cube 2_v4 (Autodesk Fusion 360 design; units mm, degrees)
Autodesk Fusion 360 part; units mm, degrees
(part 1 of 2)
sketch "b  stock" plane through (0, 0, 0) normal (0, 0, 1) x (1, 0, 0)
  line L0 (0, 0) -> (50, 0)
  line L1 (50, 0) -> (50, 304.8)
  line L2 (50, 304.8) -> (0, 304.8)
  line L3 (0, 304.8) -> (0, 0)
extrude "b  stock body extrude" add sketch "b  stock" along normal blind 3.175 makes body 1
sketch "b  layout" plane through (0, 0, 0) normal (0, 0, 1) x (1, 0, 0)
  line L0 (0, 0) -> (48, 0)
  line L1 (48, 0) -> (48, 48)
  line L2 (48, 48) -> (0, 48)
  line L3 (0, 48) -> (0, 0)
  line L4 (0, 50.01) -> (48, 50.01)
  line L5 (48, 50.01) -> (48, 98.01)
  line L6 (48, 98.01) -> (0, 98.01)
  line L7 (0, 98.01) -> (0, 50.01)
  line L8 (0, 100.02) -> (48, 100.02)
  line L9 (48, 100.02) -> (48, 148.02)
  line L10 (48, 148.02) -> (0, 148.02)
  line L11 (0, 148.02) -> (0, 100.02)
  line L12 (0, 150.03) -> (48, 150.03)
  line L13 (48, 150.03) -> (48, 198.03)
  line L14 (48, 198.03) -> (0, 198.03)
  line L15 (0, 198.03) -> (0, 150.03)
  line L16 (0, 200.04) -> (48, 200.04)
  line L17 (48, 200.04) -> (48, 248.04)
  line L18 (48, 248.04) -> (0, 248.04)
  line L19 (0, 248.04) -> (0, 200.04)
  line L20 (0, 250.05) -> (48, 250.05)
  line L21 (48, 250.05) -> (48, 298.05)
  line L22 (48, 298.05) -> (0, 298.05)
  line L23 (0, 298.05) -> (0, 250.05)
sketch "b top lines" plane through (0, 0, 0) normal (0, 0, 1) x (1, 0, 0)
  line L0 (0, 0) -> (9.1, 0)
  line L1 (9.1, 0) -> (9.1, 3.175)
  line L2 (9.1, 3.175) -> (18.9, 3.175)
  line L3 (18.9, 3.175) -> (18.9, 0)
  line L4 (18.9, 0) -> (29.1, 0)
  line L5 (29.1, 0) -> (29.1, 3.175)
  line L6 (29.1, 3.175) -> (38.9, 3.175)
  line L7 (38.9, 3.175) -> (38.9, 0)
  line L8 (38.9, 0) -> (48, 0)
  line L9 (48, 0) -> (48, 9.1)
  line L10 (48, 9.1) -> (44.825, 9.1)
  line L11 (44.825, 9.1) -> (44.825, 18.9)
  line L12 (44.825, 18.9) -> (48, 18.9)
  line L13 (48, 18.9) -> (48, 29.1)
  line L14 (48, 29.1) -> (44.825, 29.1)
  line L15 (44.825, 29.1) -> (44.825, 38.9)
  line L16 (44.825, 38.9) -> (48, 38.9)
  line L17 (48, 38.9) -> (48, 48)
  line L18 (0, 48) -> (9.1, 48)
  line L19 (9.1, 48) -> (9.1, 44.825)
  line L20 (9.1, 44.825) -> (18.9, 44.825)
  line L21 (18.9, 44.825) -> (18.9, 48)
  line L22 (18.9, 48) -> (29.1, 48)
  line L23 (29.1, 48) -> (29.1, 44.825)
  line L24 (29.1, 44.825) -> (38.9, 44.825)
  line L25 (38.9, 44.825) -> (38.9, 48)
  line L26 (38.9, 48) -> (48, 48)
  line L27 (0, 0) -> (0, 9.1)
  line L28 (0, 9.1) -> (3.175, 9.1)
  line L29 (3.175, 9.1) -> (3.175, 18.9)
  line L30 (3.175, 18.9) -> (0, 18.9)
  line L31 (0, 18.9) -> (0, 29.1)
  line L32 (0, 29.1) -> (3.175, 29.1)
  line L33 (3.175, 29.1) -> (3.175, 38.9)
  line L34 (3.175, 38.9) -> (0, 38.9)
  line L35 (0, 38.9) -> (0, 48)
  dimension "d15" = 9.1
  dimension "d16" = 3.175
  dimension "d17" = 9.8
  dimension "d18" = 3.175
  dimension "d19" = 10.2
  dimension "d20" = 3.175
  dimension "d21" = 9.8
  dimension "d22" = 3.175
  dimension "d23" = 9.1
  dimension "d28" = 9.1
  dimension "d29" = 3.175
  dimension "d30" = 9.8
  dimension "d31" = 3.175
  dimension "d32" = 10.2
  dimension "d33" = 3.175
  dimension "d34" = 9.8
  dimension "d35" = 3.175
  dimension "d36" = 9.1
  dimension "d41" = 9.1
  dimension "d42" = 3.175
  dimension "d43" = 9.8
  dimension "d44" = 3.175
  dimension "d45" = 10.2
  dimension "d46" = 3.175
  dimension "d47" = 9.8
  dimension "d48" = 3.175
  dimension "d49" = 9.1
  dimension "d54" = 9.1
  dimension "d55" = 3.175
  dimension "d56" = 9.8
  dimension "d57" = 3.175
  dimension "d58" = 10.2
  dimension "d59" = 3.175
  dimension "d60" = 9.8
  dimension "d61" = 3.175
  dimension "d62" = 9.1
  constraint horizontal L0
  constraint vertical L1
  constraint horizontal L2
  constraint vertical L3
  constraint horizontal L4
  constraint vertical L5
  constraint horizontal L6
  constraint vertical L7
  constraint horizontal L8
  constraint vertical L9
  constraint horizontal L10
  constraint vertical L11
  constraint horizontal L12
  constraint vertical L13
  constraint horizontal L14
  constraint vertical L15
  constraint horizontal L16
  constraint vertical L17
  constraint horizontal L18
  constraint vertical L19
  constraint horizontal L20
  constraint vertical L21
  constraint horizontal L22
  constraint vertical L23
  constraint horizontal L24
  constraint vertical L25
  constraint horizontal L26
  constraint vertical L27
  constraint horizontal L28
  constraint vertical L29
  constraint horizontal L30
  constraint vertical L31
  constraint horizontal L32
  constraint vertical L33
  constraint horizontal L34
  constraint vertical L35
  measures "d15" distance of L0.start L0.end
  measures "d16" distance of L0.end L1.end
  measures "d17" distance of L1.end L2.end
  measures "d18" distance of L2.end L3.end
  measures "d19" distance of L3.end L4.end
  measures "d20" distance of L4.end L5.end
  measures "d21" distance of L5.end L6.end
  measures "d22" distance of L6.end L7.end
  measures "d23" distance of L7.end L8.end
  measures "d28" distance of L8.end L9.end
  measures "d29" distance of L9.end L10.end
  measures "d30" distance of L10.end L11.end
  measures "d31" distance of L11.end L12.end
  measures "d32" distance of L12.end L13.end
  measures "d33" distance of L13.end L14.end
  measures "d34" distance of L14.end L15.end
  measures "d35" distance of L15.end L16.end
  measures "d36" distance of L16.end L17.end
  measures "d41" distance of L18.start L18.end
  measures "d42" distance of L18.end L19.end
  measures "d43" distance of L19.end L20.end
  measures "d44" distance of L20.end L21.end
  measures "d45" distance of L21.end L22.end
  measures "d46" distance of L22.end L23.end
  measures "d47" distance of L23.end L24.end
  measures "d48" distance of L24.end L25.end
  measures "d49" distance of L17.end L25.end
  measures "d54" distance of L0.start L27.end
  measures "d55" distance of L27.end L28.end
  measures "d56" distance of L28.end L29.end
  measures "d57" distance of L29.end L30.end
  measures "d58" distance of L30.end L31.end
  measures "d59" distance of L31.end L32.end
  measures "d60" distance of L32.end L33.end
  measures "d61" distance of L33.end L34.end
  measures "d62" distance of L18.start L34.end
sketch "b top circles" plane through (0, 0, 0) normal (0, 0, 1) x (1, 0, 0)
  line L0 (0, 0) -> (48, 0)
  line L1 (48, 0) -> (48, 48)
  line L2 (48, 48) -> (0, 48)
  line L3 (0, 48) -> (0, 0)
  circle A0 centre (9.6906, 2.3644) radius 1.005
  circle A1 centre (18.3094, 2.3644) radius 1.005
  circle A2 centre (29.6906, 2.3644) radius 1.005
  circle A3 centre (38.3094, 2.3644) radius 1.005
  circle A4 centre (45.6356, 9.6906) radius 1.005
  circle A5 centre (45.6356, 18.3094) radius 1.005
  circle A6 centre (45.6356, 29.6906) radius 1.005
  circle A7 centre (45.6356, 38.3094) radius 1.005
  circle A8 centre (9.6906, 45.6356) radius 1.005
  circle A9 centre (18.3094, 45.6356) radius 1.005
  circle A10 centre (29.6906, 45.6356) radius 1.005
  circle A11 centre (38.3094, 45.6356) radius 1.005
  circle A12 centre (2.3644, 9.6906) radius 1.005
  circle A13 centre (2.3644, 18.3094) radius 1.005
  circle A14 centre (2.3644, 29.6906) radius 1.005
  circle A15 centre (2.3644, 38.3094) radius 1.005
  dimension "d24" = 2.01
  dimension "d25" = 2.01
  dimension "d26" = 2.01
  dimension "d27" = 2.01
  dimension "d37" = 2.01
  dimension "d38" = 2.01
  dimension "d39" = 2.01
  dimension "d40" = 2.01
  dimension "d50" = 2.01
  dimension "d51" = 2.01
  dimension "d52" = 2.01
  dimension "d53" = 2.01
  dimension "d63" = 2.01
  dimension "d64" = 2.01
  dimension "d65" = 2.01
  dimension "d66" = 2.01
  measures "d24" diameter of A0
  measures "d25" diameter of A1
  measures "d26" diameter of A2
  measures "d27" diameter of A3
  measures "d37" diameter of A4
  measures "d38" diameter of A5
  measures "d39" diameter of A6
  measures "d40" diameter of A7
  measures "d50" diameter of A8
  measures "d51" diameter of A9
  measures "d52" diameter of A10
  measures "d53" diameter of A11
  measures "d63" diameter of A12
  measures "d64" diameter of A13
  measures "d65" diameter of A14
  measures "d66" diameter of A15
extrude "b top lines body extrude" add sketch "b top lines" along normal blind 3.175 separate body makes body 2
extrude "b top circles extrude" add sketch "b top circles" along normal blind 3.175 separate body makes body 3
combine "b top lines final combine feature" operation intersect target body 2 tool bodies 3
sketch "b front lines" plane through (0, 0, 0) normal (0, 0, 1) x (1, 0, 0)
  line L0 (3.175, 53.185) -> (8.9, 53.185)
  line L1 (8.9, 53.185) -> (8.9, 50.01)
  line L2 (8.9, 50.01) -> (19.1, 50.01)
  line L3 (19.1, 50.01) -> (19.1, 53.185)
  line L4 (19.1, 53.185) -> (28.9, 53.185)
  line L5 (28.9, 53.185) -> (28.9, 50.01)
  line L6 (28.9, 50.01) -> (39.1, 50.01)
  line L7 (39.1, 50.01) -> (39.1, 53.185)
  line L8 (39.1, 53.185) -> (44.825, 53.185)
  line L9 (44.825, 53.185) -> (44.825, 58.91)
  line L10 (44.825, 58.91) -> (48, 58.91)
  line L11 (48, 58.91) -> (48, 69.11)
  line L12 (48, 69.11) -> (44.825, 69.11)
  line L13 (44.825, 69.11) -> (44.825, 78.91)
  line L14 (44.825, 78.91) -> (48, 78.91)
  line L15 (48, 78.91) -> (48, 89.11)
  line L16 (48, 89.11) -> (44.825, 89.11)
  line L17 (44.825, 89.11) -> (44.825, 94.835)
  line L18 (3.175, 94.835) -> (8.9, 94.835)
  line L19 (8.9, 94.835) -> (8.9, 98.01)
  line L20 (8.9, 98.01) -> (19.1, 98.01)
  line L21 (19.1, 98.01) -> (19.1, 94.835)
  line L22 (19.1, 94.835) -> (28.9, 94.835)
  line L23 (28.9, 94.835) -> (28.9, 98.01)
  line L24 (28.9, 98.01) -> (39.1, 98.01)
  line L25 (39.1, 98.01) -> (39.1, 94.835)
  line L26 (39.1, 94.835) -> (44.825, 94.835)
  line L27 (3.175, 53.185) -> (3.175, 58.91)
  line L28 (3.175, 58.91) -> (0, 58.91)
  line L29 (0, 58.91) -> (0, 69.11)
  line L30 (0, 69.11) -> (3.175, 69.11)
  line L31 (3.175, 69.11) -> (3.175, 78.91)
  line L32 (3.175, 78.91) -> (0, 78.91)
  line L33 (0, 78.91) -> (0, 89.11)
  line L34 (0, 89.11) -> (3.175, 89.11)
  line L35 (3.175, 89.11) -> (3.175, 94.835)
  dimension "d71" = 5.725
  dimension "d72" = 3.175
  dimension "d73" = 10.2
  dimension "d74" = 3.175
  dimension "d75" = 9.8
  dimension "d76" = 3.175
  dimension "d77" = 10.2
  dimension "d78" = 3.175
  dimension "d79" = 5.725
  dimension "d84" = 5.725
  dimension "d85" = 3.175
  dimension "d86" = 10.2
  dimension "d87" = 3.175
  dimension "d88" = 9.8
  dimension "d89" = 3.175
  dimension "d90" = 10.2
  dimension "d91" = 3.175
  dimension "d92" = 5.725
  dimension "d97" = 5.725
  dimension "d98" = 3.175
  dimension "d99" = 10.2
  dimension "d100" = 3.175
  dimension "d101" = 9.8
  dimension "d102" = 3.175
  dimension "d103" = 10.2
  dimension "d104" = 3.175
  dimension "d105" = 5.725
  dimension "d110" = 5.725
  dimension "d111" = 3.175
  dimension "d112" = 10.2
  dimension "d113" = 3.175
  dimension "d114" = 9.8
  dimension "d115" = 3.175
  dimension "d116" = 10.2
  dimension "d117" = 3.175
  dimension "d118" = 5.725
  constraint horizontal L0
  constraint vertical L1
  constraint horizontal L2
  constraint vertical L3
  constraint horizontal L4
  constraint vertical L5
  constraint horizontal L6
  constraint vertical L7
  constraint horizontal L8
  constraint vertical L9
  constraint horizontal L10
  constraint vertical L11
  constraint horizontal L12
  constraint vertical L13
  constraint horizontal L14
  constraint vertical L15
  constraint horizontal L16
  constraint vertical L17
  constraint horizontal L18
  constraint vertical L19
  constraint horizontal L20
  constraint vertical L21
  constraint horizontal L22
  constraint vertical L23
  constraint horizontal L24
  constraint vertical L25
  constraint horizontal L26
  constraint vertical L27
  constraint horizontal L28
  constraint vertical L29
  constraint horizontal L30
  constraint vertical L31
  constraint horizontal L32
  constraint vertical L33
  constraint horizontal L34
  constraint vertical L35
  measures "d71" distance of L0.start L0.end
  measures "d72" distance of L0.end L1.end
  measures "d73" distance of L1.end L2.end
  measures "d74" distance of L2.end L3.end
  measures "d75" distance of L3.end L4.end
  measures "d76" distance of L4.end L5.end
  measures "d77" distance of L5.end L6.end
  measures "d78" distance of L6.end L7.end
  measures "d79" distance of L7.end L8.end
  measures "d84" distance of L8.end L9.end
  measures "d85" distance of L9.end L10.end
  measures "d86" distance of L10.end L11.end
  measures "d87" distance of L11.end L12.end
  measures "d88" distance of L12.end L13.end
  measures "d89" distance of L13.end L14.end
  measures "d90" distance of L14.end L15.end
  measures "d91" distance of L15.end L16.end
  measures "d92" distance of L16.end L17.end
  measures "d97" distance of L18.start L18.end
  measures "d98" distance of L18.end L19.end
  measures "d99" distance of L19.end L20.end
  measures "d100" distance of L20.end L21.end
  measures "d101" distance of L21.end L22.end
  measures "d102" distance of L22.end L23.end
  measures "d103" distance of L23.end L24.end
  measures "d104" distance of L24.end L25.end
  measures "d105" distance of L17.end L25.end
  measures "d110" distance of L0.start L27.end
  measures "d111" distance of L27.end L28.end
  measures "d112" distance of L28.end L29.end
  measures "d113" distance of L29.end L30.end
  measures "d114" distance of L30.end L31.end
  measures "d115" distance of L31.end L32.end
  measures "d116" distance of L32.end L33.end
  measures "d117" distance of L33.end L34.end
  measures "d118" distance of L18.start L34.end
sketch "b front circles" plane through (0, 0, 0) normal (0, 0, 1) x (1, 0, 0)
  line L0 (0, 50.01) -> (48, 50.01)
  line L1 (48, 50.01) -> (48, 98.01)
  line L2 (48, 98.01) -> (0, 98.01)
  line L3 (0, 98.01) -> (0, 50.01)
  circle A0 centre (8.3094, 52.3744) radius 1.005
  circle A1 centre (19.6906, 52.3744) radius 1.005
  circle A2 centre (28.3094, 52.3744) radius 1.005
  circle A3 centre (39.6906, 52.3744) radius 1.005
  circle A4 centre (45.6356, 58.3194) radius 1.005
  circle A5 centre (45.6356, 69.7006) radius 1.005
  circle A6 centre (45.6356, 78.3194) radius 1.005
  circle A7 centre (45.6356, 89.7006) radius 1.005
  circle A8 centre (8.3094, 95.6456) radius 1.005
  circle A9 centre (19.6906, 95.6456) radius 1.005
  circle A10 centre (28.3094, 95.6456) radius 1.005
  circle A11 centre (39.6906, 95.6456) radius 1.005
  circle A12 centre (2.3644, 58.3194) radius 1.005
  circle A13 centre (2.3644, 69.7006) radius 1.005
  circle A14 centre (2.3644, 78.3194) radius 1.005
  circle A15 centre (2.3644, 89.7006) radius 1.005
  dimension "d80" = 2.01
  dimension "d81" = 2.01
  dimension "d82" = 2.01
  dimension "d83" = 2.01
  dimension "d93" = 2.01
  dimension "d94" = 2.01
  dimension "d95" = 2.01
  dimension "d96" = 2.01
  dimension "d106" = 2.01
  dimension "d107" = 2.01
  dimension "d108" = 2.01
  dimension "d109" = 2.01
  dimension "d119" = 2.01
  dimension "d120" = 2.01
  dimension "d121" = 2.01
  dimension "d122" = 2.01
  measures "d80" diameter of A0
  measures "d81" diameter of A1
  measures "d82" diameter of A2
  measures "d83" diameter of A3
  measures "d93" diameter of A4
  measures "d94" diameter of A5
  measures "d95" diameter of A6
  measures "d96" diameter of A7
  measures "d106" diameter of A8
  measures "d107" diameter of A9
  measures "d108" diameter of A10
  measures "d109" diameter of A11
  measures "d119" diameter of A12
  measures "d120" diameter of A13
  measures "d121" diameter of A14
  measures "d122" diameter of A15
extrude "b front lines body extrude" add sketch "b front lines" along normal blind 3.175 separate body makes body 4
extrude "b front circles extrude" add sketch "b front circles" along normal blind 3.175 separate body makes body 5
combine "b front lines final combine feature" operation intersect target body 4 tool bodies 5
sketch "b back lines" plane through (0, 0, 0) normal (0, 0, 1) x (1, 0, 0)
  line L0 (3.175, 103.195) -> (8.9, 103.195)
  line L1 (8.9, 103.195) -> (8.9, 100.02)
  line L2 (8.9, 100.02) -> (19.1, 100.02)
  line L3 (19.1, 100.02) -> (19.1, 103.195)
  line L4 (19.1, 103.195) -> (28.9, 103.195)
  line L5 (28.9, 103.195) -> (28.9, 100.02)
  line L6 (28.9, 100.02) -> (39.1, 100.02)
  line L7 (39.1, 100.02) -> (39.1, 103.195)
  line L8 (39.1, 103.195) -> (44.825, 103.195)
  line L9 (44.825, 103.195) -> (44.825, 108.92)
  line L10 (44.825, 108.92) -> (48, 108.92)
  line L11 (48, 108.92) -> (48, 119.12)
  line L12 (48, 119.12) -> (44.825, 119.12)
  line L13 (44.825, 119.12) -> (44.825, 128.92)
  line L14 (44.825, 128.92) -> (48, 128.92)
  line L15 (48, 128.92) -> (48, 139.12)
  line L16 (48, 139.12) -> (44.825, 139.12)
  line L17 (44.825, 139.12) -> (44.825, 144.845)
  line L18 (3.175, 144.845) -> (8.9, 144.845)
  line L19 (8.9, 144.845) -> (8.9, 148.02)
  line L20 (8.9, 148.02) -> (19.1, 148.02)
  line L21 (19.1, 148.02) -> (19.1, 144.845)
  line L22 (19.1, 144.845) -> (28.9, 144.845)
  line L23 (28.9, 144.845) -> (28.9, 148.02)
  line L24 (28.9, 148.02) -> (39.1, 148.02)
  line L25 (39.1, 148.02) -> (39.1, 144.845)
  line L26 (39.1, 144.845) -> (44.825, 144.845)
  line L27 (3.175, 103.195) -> (3.175, 108.92)
  line L28 (3.175, 108.92) -> (0, 108.92)
  line L29 (0, 108.92) -> (0, 119.12)
  line L30 (0, 119.12) -> (3.175, 119.12)
  line L31 (3.175, 119.12) -> (3.175, 128.92)
  line L32 (3.175, 128.92) -> (0, 128.92)
  line L33 (0, 128.92) -> (0, 139.12)
  line L34 (0, 139.12) -> (3.175, 139.12)
  line L35 (3.175, 139.12) -> (3.175, 144.845)
  dimension "d127" = 5.725
  dimension "d128" = 3.175
  dimension "d129" = 10.2
  dimension "d130" = 3.175
  dimension "d131" = 9.8
  dimension "d132" = 3.175
  dimension "d133" = 10.2
  dimension "d134" = 3.175
  dimension "d135" = 5.725
  dimension "d140" = 5.725
  dimension "d141" = 3.175
  dimension "d142" = 10.2
  dimension "d143" = 3.175
  dimension "d144" = 9.8
  dimension "d145" = 3.175
  dimension "d146" = 10.2
  dimension "d147" = 3.175
  dimension "d148" = 5.725
  dimension "d153" = 5.725
  dimension "d154" = 3.175
  dimension "d155" = 10.2
  dimension "d156" = 3.175
  dimension "d157" = 9.8
  dimension "d158" = 3.175
  dimension "d159" = 10.2
  dimension "d160" = 3.175
  dimension "d161" = 5.725
  dimension "d166" = 5.725
  dimension "d167" = 3.175
  dimension "d168" = 10.2
  dimension "d169" = 3.175
  dimension "d170" = 9.8
  dimension "d171" = 3.175
  dimension "d172" = 10.2
  dimension "d173" = 3.175
  dimension "d174" = 5.725
  constraint horizontal L0
  constraint vertical L1
  constraint horizontal L2
  constraint vertical L3
  constraint horizontal L4
  constraint vertical L5
  constraint horizontal L6
  constraint vertical L7
  constraint horizontal L8
  constraint vertical L9
  constraint horizontal L10
  constraint vertical L11
  constraint horizontal L12
  constraint vertical L13
  constraint horizontal L14
  constraint vertical L15
  constraint horizontal L16
  constraint vertical L17
  constraint horizontal L18
  constraint vertical L19
  constraint horizontal L20
  constraint vertical L21
  constraint horizontal L22
  constraint vertical L23
  constraint horizontal L24
  constraint vertical L25
  constraint horizontal L26
  constraint vertical L27
  constraint horizontal L28
  constraint vertical L29
  constraint horizontal L30
  constraint vertical L31
  constraint horizontal L32
  constraint vertical L33
  constraint horizontal L34
  constraint vertical L35
  measures "d127" distance of L0.start L0.end
  measures "d128" distance of L0.end L1.end
  measures "d129" distance of L1.end L2.end
  measures "d130" distance of L2.end L3.end
  measures "d131" distance of L3.end L4.end
  measures "d132" distance of L4.end L5.end
  measures "d133" distance of L5.end L6.end
  measures "d134" distance of L6.end L7.end
  measures "d135" distance of L7.end L8.end
  measures "d140" distance of L8.end L9.end
  measures "d141" distance of L9.end L10.end
  measures "d142" distance of L10.end L11.end
  measures "d143" distance of L11.end L12.end
  measures "d144" distance of L12.end L13.end
  measures "d145" distance of L13.end L14.end
  measures "d146" distance of L14.end L15.end
  measures "d147" distance of L15.end L16.end
  measures "d148" distance of L16.end L17.end
  measures "d153" distance of L18.start L18.end
  measures "d154" distance of L18.end L19.end
  measures "d155" distance of L19.end L20.end
  measures "d156" distance of L20.end L21.end
  measures "d157" distance of L21.end L22.end
  measures "d158" distance of L22.end L23.end
  measures "d159" distance of L23.end L24.end
  measures "d160" distance of L24.end L25.end
  measures "d161" distance of L17.end L25.end
  measures "d166" distance of L0.start L27.end
  measures "d167" distance of L27.end L28.end
  measures "d168" distance of L28.end L29.end
  measures "d169" distance of L29.end L30.end
  measures "d170" distance of L30.end L31.end
  measures "d171" distance of L31.end L32.end
  measures "d172" distance of L32.end L33.end
  measures "d173" distance of L33.end L34.end
  measures "d174" distance of L18.start L34.end
sketch "b back circles" plane through (0, 0, 0) normal (0, 0, 1) x (1, 0, 0)
  line L0 (0, 100.02) -> (48, 100.02)
  line L1 (48, 100.02) -> (48, 148.02)
  line L2 (48, 148.02) -> (0, 148.02)
  line L3 (0, 148.02) -> (0, 100.02)
  circle A0 centre (8.3094, 102.3844) radius 1.005
  circle A1 centre (19.6906, 102.3844) radius 1.005
  circle A2 centre (28.3094, 102.3844) radius 1.005
  circle A3 centre (39.6906, 102.3844) radius 1.005
  circle A4 centre (45.6356, 108.3294) radius 1.005
  circle A5 centre (45.6356, 119.7106) radius 1.005
  circle A6 centre (45.6356, 128.3294) radius 1.005
  circle A7 centre (45.6356, 139.7106) radius 1.005
  circle A8 centre (8.3094, 145.6556) radius 1.005
  circle A9 centre (19.6906, 145.6556) radius 1.005
  circle A10 centre (28.3094, 145.6556) radius 1.005
  circle A11 centre (39.6906, 145.6556) radius 1.005
  circle A12 centre (2.3644, 108.3294) radius 1.005
  circle A13 centre (2.3644, 119.7106) radius 1.005
  circle A14 centre (2.3644, 128.3294) radius 1.005
  circle A15 centre (2.3644, 139.7106) radius 1.005
  dimension "d136" = 2.01
  dimension "d137" = 2.01
  dimension "d138" = 2.01
  dimension "d139" = 2.01
  dimension "d149" = 2.01
  dimension "d150" = 2.01
  dimension "d151" = 2.01
  dimension "d152" = 2.01
  dimension "d162" = 2.01
  dimension "d163" = 2.01
  dimension "d164" = 2.01
  dimension "d165" = 2.01
  dimension "d175" = 2.01
  dimension "d176" = 2.01
  dimension "d177" = 2.01
  dimension "d178" = 2.01
  measures "d136" diameter of A0
  measures "d137" diameter of A1
  measures "d138" diameter of A2
  measures "d139" diameter of A3
  measures "d149" diameter of A4
  measures "d150" diameter of A5
  measures "d151" diameter of A6
  measures "d152" diameter of A7
  measures "d162" diameter of A8
  measures "d163" diameter of A9
  measures "d164" diameter of A10
  measures "d165" diameter of A11
  measures "d175" diameter of A12
  measures "d176" diameter of A13
  measures "d177" diameter of A14
  measures "d178" diameter of A15
extrude "b back lines body extrude" add sketch "b back lines" along normal blind 3.175 separate body makes body 6
extrude "b back circles extrude" add sketch "b back circles" along normal blind 3.175 separate body makes body 7
combine "b back lines final combine feature" operation intersect target body 6 tool bodies 7
sketch "b left lines" plane through (0, 0, 0) normal (0, 0, 1) x (1, 0, 0)
  line L0 (3.175, 150.03) -> (9.1, 150.03)
  line L1 (9.1, 150.03) -> (9.1, 153.205)
  line L2 (9.1, 153.205) -> (18.9, 153.205)
  line L3 (18.9, 153.205) -> (18.9, 150.03)
  line L4 (18.9, 150.03) -> (29.1, 150.03)
  line L5 (29.1, 150.03) -> (29.1, 153.205)
  line L6 (29.1, 153.205) -> (38.9, 153.205)
  line L7 (38.9, 153.205) -> (38.9, 150.03)
  line L8 (38.9, 150.03) -> (44.825, 150.03)
  line L9 (44.825, 150.03) -> (44.825, 158.93)
  line L10 (44.825, 158.93) -> (48, 158.93)
  line L11 (48, 158.93) -> (48, 169.13)
  line L12 (48, 169.13) -> (44.825, 169.13)
  line L13 (44.825, 169.13) -> (44.825, 178.93)
  line L14 (44.825, 178.93) -> (48, 178.93)
  line L15 (48, 178.93) -> (48, 189.13)
  line L16 (48, 189.13) -> (44.825, 189.13)
  line L17 (44.825, 189.13) -> (44.825, 198.03)
  line L18 (3.175, 198.03) -> (9.1, 198.03)
  line L19 (9.1, 198.03) -> (9.1, 194.855)
  line L20 (9.1, 194.855) -> (18.9, 194.855)
  line L21 (18.9, 194.855) -> (18.9, 198.03)
  line L22 (18.9, 198.03) -> (29.1, 198.03)
  line L23 (29.1, 198.03) -> (29.1, 194.855)
  line L24 (29.1, 194.855) -> (38.9, 194.855)
  line L25 (38.9, 194.855) -> (38.9, 198.03)
  line L26 (38.9, 198.03) -> (44.825, 198.03)
  line L27 (3.175, 150.03) -> (3.175, 158.93)
  line L28 (3.175, 158.93) -> (0, 158.93)
  line L29 (0, 158.93) -> (0, 169.13)
  line L30 (0, 169.13) -> (3.175, 169.13)
  line L31 (3.175, 169.13) -> (3.175, 178.93)
  line L32 (3.175, 178.93) -> (0, 178.93)
  line L33 (0, 178.93) -> (0, 189.13)
  line L34 (0, 189.13) -> (3.175, 189.13)
  line L35 (3.175, 189.13) -> (3.175, 198.03)
  dimension "d183" = 5.925
  dimension "d184" = 3.175
  dimension "d185" = 9.8
  dimension "d186" = 3.175
  dimension "d187" = 10.2
  dimension "d188" = 3.175
  dimension "d189" = 9.8
  dimension "d190" = 3.175
  dimension "d191" = 5.925
  dimension "d196" = 8.9
  dimension "d197" = 3.175
  dimension "d198" = 10.2
  dimension "d199" = 3.175
  dimension "d200" = 9.8
  dimension "d201" = 3.175
  dimension "d202" = 10.2
  dimension "d203" = 3.175
  dimension "d204" = 8.9
  dimension "d209" = 5.925
  dimension "d210" = 3.175
  dimension "d211" = 9.8
  dimension "d212" = 3.175
  dimension "d213" = 10.2
  dimension "d214" = 3.175
  dimension "d215" = 9.8
  dimension "d216" = 3.175
  dimension "d217" = 5.925
  dimension "d222" = 8.9
  dimension "d223" = 3.175
  dimension "d224" = 10.2
  dimension "d225" = 3.175
  dimension "d226" = 9.8
  dimension "d227" = 3.175
  dimension "d228" = 10.2
  dimension "d229" = 3.175
  dimension "d230" = 8.9
  constraint horizontal L0
  constraint vertical L1
  constraint horizontal L2
  constraint vertical L3
  constraint horizontal L4
  constraint vertical L5
  constraint horizontal L6
  constraint vertical L7
  constraint horizontal L8
  constraint vertical L9
  constraint horizontal L10
  constraint vertical L11
  constraint horizontal L12
  constraint vertical L13
  constraint horizontal L14
  constraint vertical L15
  constraint horizontal L16
  constraint vertical L17
  constraint horizontal L18
  constraint vertical L19
  constraint horizontal L20
  constraint vertical L21
  constraint horizontal L22
  constraint vertical L23
  constraint horizontal L24
  constraint vertical L25
  constraint horizontal L26
  constraint vertical L27
  constraint horizontal L28
  constraint vertical L29
  constraint horizontal L30
  constraint vertical L31
  constraint horizontal L32
  constraint vertical L33
  constraint horizontal L34
  constraint vertical L35
  measures "d183" distance of L0.start L0.end
  measures "d184" distance of L0.end L1.end
  measures "d185" distance of L1.end L2.end
  measures "d186" distance of L2.end L3.end
  measures "d187" distance of L3.end L4.end
  measures "d188" distance of L4.end L5.end
  measures "d189" distance of L5.end L6.end
  measures "d190" distance of L6.end L7.end
  measures "d191" distance of L7.end L8.end
  measures "d196" distance of L8.end L9.end
  measures "d197" distance of L9.end L10.end
  measures "d198" distance of L10.end L11.end
  measures "d199" distance of L11.end L12.end
  measures "d200" distance of L12.end L13.end
  measures "d201" distance of L13.end L14.end
  measures "d202" distance of L14.end L15.end
  measures "d203" distance of L15.end L16.end
  measures "d204" distance of L16.end L17.end
  measures "d209" distance of L18.start L18.end
  measures "d210" distance of L18.end L19.end
  measures "d211" distance of L19.end L20.end
  measures "d212" distance of L20.end L21.end
  measures "d213" distance of L21.end L22.end
  measures "d214" distance of L22.end L23.end
  measures "d215" distance of L23.end L24.end
  measures "d216" distance of L24.end L25.end
  measures "d217" distance of L17.end L25.end
  measures "d222" distance of L0.start L27.end
  measures "d223" distance of L27.end L28.end
  measures "d224" distance of L28.end L29.end
  measures "d225" distance of L29.end L30.end
  measures "d226" distance of L30.end L31.end
  measures "d227" distance of L31.end L32.end
  measures "d228" distance of L32.end L33.end
  measures "d229" distance of L33.end L34.end
  measures "d230" distance of L18.start L34.end
sketch "b left circles" plane through (0, 0, 0) normal (0, 0, 1) x (1, 0, 0)
  line L0 (0, 150.03) -> (48, 150.03)
  line L1 (48, 150.03) -> (48, 198.03)
  line L2 (48, 198.03) -> (0, 198.03)
  line L3 (0, 198.03) -> (0, 150.03)
  circle A0 centre (9.6906, 152.3944) radius 1.005
  circle A1 centre (18.3094, 152.3944) radius 1.005
  circle A2 centre (29.6906, 152.3944) radius 1.005
  circle A3 centre (38.3094, 152.3944) radius 1.005
  circle A4 centre (45.6356, 158.3394) radius 1.005
  circle A5 centre (45.6356, 169.7206) radius 1.005
  circle A6 centre (45.6356, 178.3394) radius 1.005
  circle A7 centre (45.6356, 189.7206) radius 1.005
  circle A8 centre (9.6906, 195.6656) radius 1.005
  circle A9 centre (18.3094, 195.6656) radius 1.005
  circle A10 centre (29.6906, 195.6656) radius 1.005
  circle A11 centre (38.3094, 195.6656) radius 1.005
  circle A12 centre (2.3644, 158.3394) radius 1.005
  circle A13 centre (2.3644, 169.7206) radius 1.005
  circle A14 centre (2.3644, 178.3394) radius 1.005
  circle A15 centre (2.3644, 189.7206) radius 1.005
  dimension "d192" = 2.01
  dimension "d193" = 2.01
  dimension "d194" = 2.01
  dimension "d195" = 2.01
  dimension "d205" = 2.01
  dimension "d206" = 2.01
  dimension "d207" = 2.01
  dimension "d208" = 2.01
  dimension "d218" = 2.01
  dimension "d219" = 2.01
  dimension "d220" = 2.01
  dimension "d221" = 2.01
  dimension "d231" = 2.01
  dimension "d232" = 2.01
  dimension "d233" = 2.01
  dimension "d234" = 2.01
  measures "d192" diameter of A0
  measures "d193" diameter of A1
  measures "d194" diameter of A2
  measures "d195" diameter of A3
  measures "d205" diameter of A4
  measures "d206" diameter of A5
  measures "d207" diameter of A6
  measures "d208" diameter of A7
  measures "d218" diameter of A8
  measures "d219" diameter of A9
  measures "d220" diameter of A10
  measures "d221" diameter of A11
  measures "d231" diameter of A12
  measures "d232" diameter of A13
  measures "d233" diameter of A14
  measures "d234" diameter of A15
extrude "b left lines body extrude" add sketch "b left lines" along normal blind 3.175 separate body makes body 8
extrude "b left circles extrude" add sketch "b left circles" along normal blind 3.175 separate body makes body 9
combine "b left lines final combine feature" operation intersect target body 8 tool bodies 9
sketch "b right lines" plane through (0, 0, 0) normal (0, 0, 1) x (1, 0, 0)
  line L0 (3.175, 200.04) -> (9.1, 200.04)
  line L1 (9.1, 200.04) -> (9.1, 203.215)
  line L2 (9.1, 203.215) -> (18.9, 203.215)
  line L3 (18.9, 203.215) -> (18.9, 200.04)
  line L4 (18.9, 200.04) -> (29.1, 200.04)
  line L5 (29.1, 200.04) -> (29.1, 203.215)
  line L6 (29.1, 203.215) -> (38.9, 203.215)
  line L7 (38.9, 203.215) -> (38.9, 200.04)
  line L8 (38.9, 200.04) -> (44.825, 200.04)
  line L9 (44.825, 200.04) -> (44.825, 208.94)
  line L10 (44.825, 208.94) -> (48, 208.94)
  line L11 (48, 208.94) -> (48, 219.14)
  line L12 (48, 219.14) -> (44.825, 219.14)
  line L13 (44.825, 219.14) -> (44.825, 228.94)
  line L14 (44.825, 228.94) -> (48, 228.94)
  line L15 (48, 228.94) -> (48, 239.14)
  line L16 (48, 239.14) -> (44.825, 239.14)
  line L17 (44.825, 239.14) -> (44.825, 248.04)
  line L18 (3.175, 248.04) -> (9.1, 248.04)
  line L19 (9.1, 248.04) -> (9.1, 244.865)
  line L20 (9.1, 244.865) -> (18.9, 244.865)
  line L21 (18.9, 244.865) -> (18.9, 248.04)
  line L22 (18.9, 248.04) -> (29.1, 248.04)
  line L23 (29.1, 248.04) -> (29.1, 244.865)
  line L24 (29.1, 244.865) -> (38.9, 244.865)
  line L25 (38.9, 244.865) -> (38.9, 248.04)
  line L26 (38.9, 248.04) -> (44.825, 248.04)
  line L27 (3.175, 200.04) -> (3.175, 208.94)
  line L28 (3.175, 208.94) -> (0, 208.94)
  line L29 (0, 208.94) -> (0, 219.14)
  line L30 (0, 219.14) -> (3.175, 219.14)
  line L31 (3.175, 219.14) -> (3.175, 228.94)
  line L32 (3.175, 228.94) -> (0, 228.94)
  line L33 (0, 228.94) -> (0, 239.14)
  line L34 (0, 239.14) -> (3.175, 239.14)
  line L35 (3.175, 239.14) -> (3.175, 248.04)
  dimension "d239" = 5.925
  dimension "d240" = 3.175
  dimension "d241" = 9.8
  dimension "d242" = 3.175
  dimension "d243" = 10.2
  dimension "d244" = 3.175
  dimension "d245" = 9.8
  dimension "d246" = 3.175
  dimension "d247" = 5.925
  dimension "d252" = 8.9
  dimension "d253" = 3.175
  dimension "d254" = 10.2
  dimension "d255" = 3.175
  dimension "d256" = 9.8
  dimension "d257" = 3.175
  dimension "d258" = 10.2
  dimension "d259" = 3.175
  dimension "d260" = 8.9
  dimension "d265" = 5.925
  dimension "d266" = 3.175
  dimension "d267" = 9.8
  dimension "d268" = 3.175
  dimension "d269" = 10.2
  dimension "d270" = 3.175
  dimension "d271" = 9.8
  dimension "d272" = 3.175
  dimension "d273" = 5.925
  dimension "d278" = 8.9
  dimension "d279" = 3.175
  dimension "d280" = 10.2
  dimension "d281" = 3.175
  dimension "d282" = 9.8
  dimension "d283" = 3.175
  dimension "d284" = 10.2
  dimension "d285" = 3.175
  dimension "d286" = 8.9
  constraint horizontal L0
  constraint vertical L1
  constraint horizontal L2
  constraint vertical L3
  constraint horizontal L4
  constraint vertical L5
  constraint horizontal L6
  constraint vertical L7
  constraint horizontal L8
  constraint vertical L9
  constraint horizontal L10
  constraint vertical L11
  constraint horizontal L12
  constraint vertical L13
  constraint horizontal L14
  constraint vertical L15
  constraint horizontal L16
  constraint vertical L17
  constraint horizontal L18
  constraint vertical L19
  constraint horizontal L20
  constraint vertical L21
  constraint horizontal L22
  constraint vertical L23
  constraint horizontal L24
  constraint vertical L25
  constraint horizontal L26
  constraint vertical L27
  constraint horizontal L28
  constraint vertical L29
  constraint horizontal L30
  constraint vertical L31
  constraint horizontal L32
  constraint vertical L33
  constraint horizontal L34
  constraint vertical L35
  measures "d239" distance of L0.start L0.end
  measures "d240" distance of L0.end L1.end
  measures "d241" distance of L1.end L2.end
  measures "d242" distance of L2.end L3.end
  measures "d243" distance of L3.end L4.end
  measures "d244" distance of L4.end L5.end
  measures "d245" distance of L5.end L6.end
  measures "d246" distance of L6.end L7.end
  measures "d247" distance of L7.end L8.end
  measures "d252" distance of L8.end L9.end
  measures "d253" distance of L9.end L10.end
  measures "d254" distance of L10.end L11.end
  measures "d255" distance of L11.end L12.end
  measures "d256" distance of L12.end L13.end
  measures "d257" distance of L13.end L14.end
  measures "d258" distance of L14.end L15.end
  measures "d259" distance of L15.end L16.end
  measures "d260" distance of L16.end L17.end
  measures "d265" distance of L18.start L18.end
  measures "d266" distance of L18.end L19.end
  measures "d267" distance of L19.end L20.end
  measures "d268" distance of L20.end L21.end
  measures "d269" distance of L21.end L22.end
  measures "d270" distance of L22.end L23.end
  measures "d271" distance of L23.end L24.end
  measures "d272" distance of L24.end L25.end
  measures "d273" distance of L17.end L25.end
  measures "d278" distance of L0.start L27.end
  measures "d279" distance of L27.end L28.end
  measures "d280" distance of L28.end L29.end
  measures "d281" distance of L29.end L30.end
  measures "d282" distance of L30.end L31.end
  measures "d283" distance of L31.end L32.end
  measures "d284" distance of L32.end L33.end
  measures "d285" distance of L33.end L34.end
  measures "d286" distance of L18.start L34.end
sketch "b right circles" plane through (0, 0, 0) normal (0, 0, 1) x (1, 0, 0)
  line L0 (0, 200.04) -> (48, 200.04)
  line L1 (48, 200.04) -> (48, 248.04)
  line L2 (48, 248.04) -> (0, 248.04)
  line L3 (0, 248.04) -> (0, 200.04)
  circle A0 centre (9.6906, 202.4044) radius 1.005
  circle A1 centre (18.3094, 202.4044) radius 1.005
  circle A2 centre (29.6906, 202.4044) radius 1.005
  circle A3 centre (38.3094, 202.4044) radius 1.005
  circle A4 centre (45.6356, 208.3494) radius 1.005
  circle A5 centre (45.6356, 219.7306) radius 1.005
  circle A6 centre (45.6356, 228.3494) radius 1.005
  circle A7 centre (45.6356, 239.7306) radius 1.005
  circle A8 centre (9.6906, 245.6756) radius 1.005
  circle A9 centre (18.3094, 245.6756) radius 1.005
  circle A10 centre (29.6906, 245.6756) radius 1.005
  circle A11 centre (38.3094, 245.6756) radius 1.005
  circle A12 centre (2.3644, 208.3494) radius 1.005
  circle A13 centre (2.3644, 219.7306) radius 1.005
  circle A14 centre (2.3644, 228.3494) radius 1.005
  circle A15 centre (2.3644, 239.7306) radius 1.005
  dimension "d248" = 2.01
  dimension "d249" = 2.01
  dimension "d250" = 2.01
  dimension "d251" = 2.01
  dimension "d261" = 2.01
  dimension "d262" = 2.01
  dimension "d263" = 2.01
  dimension "d264" = 2.01
  dimension "d274" = 2.01
  dimension "d275" = 2.01
  dimension "d276" = 2.01
  dimension "d277" = 2.01
  dimension "d287" = 2.01
  dimension "d288" = 2.01
  dimension "d289" = 2.01
  dimension "d290" = 2.01
  measures "d248" diameter of A0
  measures "d249" diameter of A1
  measures "d250" diameter of A2
  measures "d251" diameter of A3
  measures "d261" diameter of A4
  measures "d262" diameter of A5
  measures "d263" diameter of A6
  measures "d264" diameter of A7
  measures "d274" diameter of A8
  measures "d275" diameter of A9
  measures "d276" diameter of A10
  measures "d277" diameter of A11
  measures "d287" diameter of A12
  measures "d288" diameter of A13
  measures "d289" diameter of A14
  measures "d290" diameter of A15
extrude "b right lines body extrude" add sketch "b right lines" along normal blind 3.175 separate body makes body 10
extrude "b right circles extrude" add sketch "b right circles" along normal blind 3.175 separate body makes body 11
combine "b right lines final combine feature" operation intersect target body 10 tool bodies 11
sketch "b bottom lines" plane through (0, 0, 0) normal (0, 0, 1) x (1, 0, 0)
  line L0 (0, 250.05) -> (9.1, 250.05)
  line L1 (9.1, 250.05) -> (9.1, 253.225)
  line L2 (9.1, 253.225) -> (18.9, 253.225)
  line L3 (18.9, 253.225) -> (18.9, 250.05)
  line L4 (18.9, 250.05) -> (29.1, 250.05)
  line L5 (29.1, 250.05) -> (29.1, 253.225)
  line L6 (29.1, 253.225) -> (38.9, 253.225)
  line L7 (38.9, 253.225) -> (38.9, 250.05)
  line L8 (38.9, 250.05) -> (48, 250.05)
  line L9 (48, 250.05) -> (48, 259.15)
  line L10 (48, 259.15) -> (44.825, 259.15)
  line L11 (44.825, 259.15) -> (44.825, 268.95)
  line L12 (44.825, 268.95) -> (48, 268.95)
  line L13 (48, 268.95) -> (48, 279.15)
  line L14 (48, 279.15) -> (44.825, 279.15)
  line L15 (44.825, 279.15) -> (44.825, 288.95)
  line L16 (44.825, 288.95) -> (48, 288.95)
  line L17 (48, 288.95) -> (48, 298.05)
  line L18 (0, 298.05) -> (9.1, 298.05)
  line L19 (9.1, 298.05) -> (9.1, 294.875)
  line L20 (9.1, 294.875) -> (18.9, 294.875)
  line L21 (18.9, 294.875) -> (18.9, 298.05)
  line L22 (18.9, 298.05) -> (29.1, 298.05)
  line L23 (29.1, 298.05) -> (29.1, 294.875)
  line L24 (29.1, 294.875) -> (38.9, 294.875)
  line L25 (38.9, 294.875) -> (38.9, 298.05)
  line L26 (38.9, 298.05) -> (48, 298.05)
  line L27 (0, 250.05) -> (0, 259.15)
  line L28 (0, 259.15) -> (3.175, 259.15)
  line L29 (3.175, 259.15) -> (3.175, 268.95)
  line L30 (3.175, 268.95) -> (0, 268.95)
  line L31 (0, 268.95) -> (0, 279.15)
  line L32 (0, 279.15) -> (3.175, 279.15)
  line L33 (3.175, 279.15) -> (3.175, 288.95)
  line L34 (3.175, 288.95) -> (0, 288.95)
  line L35 (0, 288.95) -> (0, 298.05)
  dimension "d295" = 9.1
  dimension "d296" = 3.175
  dimension "d297" = 9.8
  dimension "d298" = 3.175
  dimension "d299" = 10.2
  dimension "d300" = 3.175
  dimension "d301" = 9.8
  dimension "d302" = 3.175
  dimension "d303" = 9.1
  dimension "d308" = 9.1
  dimension "d309" = 3.175
  dimension "d310" = 9.8
  dimension "d311" = 3.175
  dimension "d312" = 10.2
  dimension "d313" = 3.175
  dimension "d314" = 9.8
  dimension "d315" = 3.175
  dimension "d316" = 9.1
  dimension "d321" = 9.1
  dimension "d322" = 3.175
  dimension "d323" = 9.8
  dimension "d324" = 3.175
  dimension "d325" = 10.2
  dimension "d326" = 3.175
  dimension "d327" = 9.8
  dimension "d328" = 3.175
  dimension "d329" = 9.1
  dimension "d334" = 9.1
  dimension "d335" = 3.175
  dimension "d336" = 9.8
  dimension "d337" = 3.175
  dimension "d338" = 10.2
  dimension "d339" = 3.175
  dimension "d340" = 9.8
  dimension "d341" = 3.175
  dimension "d342" = 9.1
  constraint horizontal L0
  constraint vertical L1
  constraint horizontal L2
  constraint vertical L3
  constraint horizontal L4
  constraint vertical L5
  constraint horizontal L6
  constraint vertical L7
  constraint horizontal L8
  constraint vertical L9
  constraint horizontal L10
  constraint vertical L11
  constraint horizontal L12
  constraint vertical L13
  constraint horizontal L14
  constraint vertical L15
  constraint horizontal L16
  constraint vertical L17
  constraint horizontal L18
  constraint vertical L19
  constraint horizontal L20
  constraint vertical L21
  constraint horizontal L22
  constraint vertical L23
  constraint horizontal L24
  constraint vertical L25
  constraint horizontal L26
  constraint vertical L27
  constraint horizontal L28
  constraint vertical L29
  constraint horizontal L30
  constraint vertical L31
  constraint horizontal L32
  constraint vertical L33
  constraint horizontal L34
  constraint vertical L35
  measures "d295" distance of L0.start L0.end
  measures "d296" distance of L0.end L1.end
  measures "d297" distance of L1.end L2.end
  measures "d298" distance of L2.end L3.end
  measures "d299" distance of L3.end L4.end
  measures "d300" distance of L4.end L5.end
  measures "d301" distance of L5.end L6.end
  measures "d302" distance of L6.end L7.end
  measures "d303" distance of L7.end L8.end
  measures "d308" distance of L8.end L9.end
  measures "d309" distance of L9.end L10.end
  measures "d310" distance of L10.end L11.end
  measures "d311" distance of L11.end L12.end
  measures "d312" distance of L12.end L13.end
  measures "d313" distance of L13.end L14.end
  measures "d314" distance of L14.end L15.end
  measures "d315" distance of L15.end L16.end
  measures "d316" distance of L16.end L17.end
  measures "d321" distance of L18.start L18.end
  measures "d322" distance of L18.end L19.end
  measures "d323" distance of L19.end L20.end
  measures "d324" distance of L20.end L21.end
  measures "d325" distance of L21.end L22.end
  measures "d326" distance of L22.end L23.end
  measures "d327" distance of L23.end L24.end
  measures "d328" distance of L24.end L25.end
  measures "d329" distance of L17.end L25.end
  measures "d334" distance of L0.start L27.end
  measures "d335" distance of L27.end L28.end
  measures "d336" distance of L28.end L29.end
  measures "d337" distance of L29.end L30.end
  measures "d338" distance of L30.end L31.end
  measures "d339" distance of L31.end L32.end
  measures "d340" distance of L32.end L33.end
  measures "d341" distance of L33.end L34.end
  measures "d342" distance of L18.start L34.end
sketch "b bottom circles" plane through (0, 0, 0) normal (0, 0, 1) x (1, 0, 0)
  line L0 (0, 250.05) -> (48, 250.05)
  line L1 (48, 250.05) -> (48, 298.05)
  line L2 (48, 298.05) -> (0, 298.05)
  line L3 (0, 298.05) -> (0, 250.05)
  circle A0 centre (9.6906, 252.4144) radius 1.005
  circle A1 centre (18.3094, 252.4144) radius 1.005
  circle A2 centre (29.6906, 252.4144) radius 1.005
  circle A3 centre (38.3094, 252.4144) radius 1.005
  circle A4 centre (45.6356, 259.7406) radius 1.005
  circle A5 centre (45.6356, 268.3594) radius 1.005
  circle A6 centre (45.6356, 279.7406) radius 1.005
  circle A7 centre (45.6356, 288.3594) radius 1.005
  circle A8 centre (9.6906, 295.6856) radius 1.005
  circle A9 centre (18.3094, 295.6856) radius 1.005
  circle A10 centre (29.6906, 295.6856) radius 1.005
  circle A11 centre (38.3094, 295.6856) radius 1.005
  circle A12 centre (2.3644, 259.7406) radius 1.005
  circle A13 centre (2.3644, 268.3594) radius 1.005
  circle A14 centre (2.3644, 279.7406) radius 1.005
  circle A15 centre (2.3644, 288.3594) radius 1.005
  dimension "d304" = 2.01
  dimension "d305" = 2.01
  dimension "d306" = 2.01
  dimension "d307" = 2.01
  dimension "d317" = 2.01
  dimension "d318" = 2.01
  dimension "d319" = 2.01
  dimension "d320" = 2.01
  dimension "d330" = 2.01
  dimension "d331" = 2.01
  dimension "d332" = 2.01
  dimension "d333" = 2.01
  dimension "d343" = 2.01
  dimension "d344" = 2.01
  dimension "d345" = 2.01
  dimension "d346" = 2.01
  measures "d304" diameter of A0
  measures "d305" diameter of A1
  measures "d306" diameter of A2
  measures "d307" diameter of A3
  measures "d317" diameter of A4
  measures "d318" diameter of A5
  measures "d319" diameter of A6
  measures "d320" diameter of A7
  measures "d330" diameter of A8
  measures "d331" diameter of A9
  measures "d332" diameter of A10
  measures "d333" diameter of A11
  measures "d343" diameter of A12
  measures "d344" diameter of A13
  measures "d345" diameter of A14
  measures "d346" diameter of A15
extrude "b bottom lines body extrude" add sketch "b bottom lines" along normal blind 3.175 separate body makes body 12
extrude "b bottom circles extrude" add sketch "b bottom circles" along normal blind 3.175 separate body makes body 13
combine "b bottom lines final combine feature" operation intersect target body 12 tool bodies 13
equation "Version_info = 0 mm" comment "1.1.0 LENGTH 48.0 DEPTH 48.0 HEIGHT 48.0 THICKNESS 3.175 TOOL_DIAMETER 2.01 TOOTH_WIDTH 10.0 KERF -0.1 DELTA_FROM_BOTTOM -0.1 STOCK_X_DIMENSION 50.0 STOCK_Y_DIMENSION 304.8 COMPONENT  REPEATS_L_TMP -1 CREATE_COMPONENTS False CREATE_BODIES 1 CREATE_EMPTY_CONTENTS False CREATE_CONSTRAINTS True CLEAR_PREVIOUSLY_GENERATED_ITEMS True JUST_CLEAR_PREVIOUSLY_GENERATED_ITEMS False CREATE_MANUFACTURING False DEBUG_JUST_ONE_PART False MANUAL_LAYOUT  SKIP_LAYOUT False JUST_BUILD_TEST False DEBUG True"
equation "Length = 48.0 mm" comment "Length (mm)"
equation "Depth = 48.0 mm" comment "Depth (mm)"
equation "Height = 48.0 mm" comment "Height (mm)"
equation "Thickness = 3.175 mm" comment "Thickness (mm)"
equation "Tool_diameter = 2.01 mm" comment "Tool Diameter (mm)"
equation "Tooth_width = 10.0 mm" comment "Target Tooth Width (mm)"
equation "Kerf = -0.1 mm" comment "Kerf (mm)- can be negative"
equation "Delta_from_bottom = -0.1 mm" comment "Additional fine adjustment of bone centers from bottom of holes(mm)- positive makes smaller bottom indents"
equation "Stock_x_dimension = 50.0 mm" comment "Stock X Dimension *"
equation "Stock_y_dimension = 304.8 mm" comment "Stock Y Dimension"
equation "Repeats_l_tmp = -1.0 mm" comment "temp hidden"
equation "d16 = Thickness"
equation "d18 = Thickness"
equation "d20 = Thickness"
equation "d22 = Thickness"
equation "d24 = Tool_diameter"
equation "d25 = Tool_diameter"
equation "d26 = Tool_diameter"
equation "d27 = Tool_diameter"
equation "d29 = Thickness"
equation "d31 = Thickness"
equation "d33 = Thickness"
equation "d35 = Thickness"
equation "d37 = Tool_diameter"
equation "d38 = Tool_diameter"
equation "d39 = Tool_diameter"
equation "d40 = Tool_diameter"
equation "d42 = Thickness"
equation "d44 = Thickness"
equation "d46 = Thickness"
equation "d48 = Thickness"
equation "d50 = Tool_diameter"
equation "d51 = Tool_diameter"
equation "d52 = Tool_diameter"
equation "d53 = Tool_diameter"
equation "d55 = Thickness"
equation "d57 = Thickness"
equation "d59 = Thickness"
equation "d61 = Thickness"
equation "d63 = Tool_diameter"
equation "d64 = Tool_diameter"
equation "d65 = Tool_diameter"
equation "d66 = Tool_diameter"
equation "d72 = Thickness"
equation "d74 = Thickness"
equation "d76 = Thickness"
equation "d78 = Thickness"
equation "d80 = Tool_diameter"
equation "d81 = Tool_diameter"
equation "d82 = Tool_diameter"
equation "d83 = Tool_diameter"
equation "d85 = Thickness"
equation "d87 = Thickness"
equation "d89 = Thickness"
equation "d91 = Thickness"
equation "d93 = Tool_diameter"
equation "d94 = Tool_diameter"
equation "d95 = Tool_diameter"
equation "d96 = Tool_diameter"
equation "d98 = Thickness"
equation "d100 = Thickness"
equation "d102 = Thickness"
equation "d104 = Thickness"
equation "d106 = Tool_diameter"
equation "d107 = Tool_diameter"
equation "d108 = Tool_diameter"
equation "d109 = Tool_diameter"
equation "d111 = Thickness"
equation "d113 = Thickness"
equation "d115 = Thickness"
equation "d117 = Thickness"
equation "d119 = Tool_diameter"
equation "d120 = Tool_diameter"
equation "d121 = Tool_diameter"
equation "d122 = Tool_diameter"
equation "d128 = Thickness"
equation "d130 = Thickness"
equation "d132 = Thickness"
equation "d134 = Thickness"
equation "d136 = Tool_diameter"
equation "d137 = Tool_diameter"
equation "d138 = Tool_diameter"
equation "d139 = Tool_diameter"
equation "d141 = Thickness"
equation "d143 = Thickness"
equation "d145 = Thickness"
equation "d147 = Thickness"
equation "d149 = Tool_diameter"
equation "d150 = Tool_diameter"
equation "d151 = Tool_diameter"
equation "d152 = Tool_diameter"
equation "d154 = Thickness"
equation "d156 = Thickness"
equation "d158 = Thickness"
equation "d160 = Thickness"
equation "d162 = Tool_diameter"
equation "d163 = Tool_diameter"
equation "d164 = Tool_diameter"
equation "d165 = Tool_diameter"